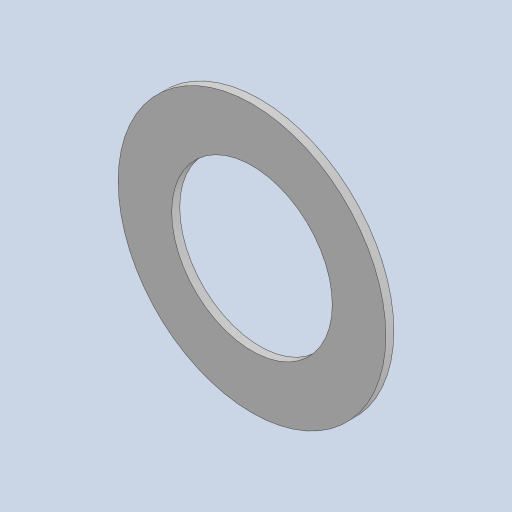
# Autodesk Inventor part: PACK-SWSJJ10-6-0_3
Saved by Autodesk Inventor 2023 (Build 270158000, 158)
## iProperties
Category: PARTsolutions
Company: MISUMI
Created: 2024-11-29
Part Number: PACK-SWSJJ10-6-0_3
Material: Generic
Catalog Web Link: www.cadenas.de
Description: SWSJJ, SWSJK, SWSPT, SWSPP, PACK-SWSJJ,PACK-SWSJK , PACK-SWSPT, PACK-SWSPP-Extra Thin Resin Washers / Sheets
Vendor: MISUMI
Document SubType Name: Modeling
Designer: psAdmin
Manufacturer: MISUMI
Mass: 0.0150796 g
Surface Area: 1.15611 cm^2
Volume: 0.0150796 cm^3
Density: 1 g/cm^3
Appearance: PSOLRGB-175-175-175
PSOL_IDENT_0: {$CADENAS_DATA/23d-libs/misumi/metric/26_washers_collars/swspt.prj},264 {VTYP=3D},{NB=PACK-SWSJJ10-6
PSOL_IDENT_1: -0.3},{LINA=PACK-SWSJJ10-6-0.3},{NN=SWSJJ, SWSJK, SWSPT, SWSPP, PACK-SWSJJ,PACK-SWSJK , PACK-SWSPT,
PSOL_IDENT_2: PACK-SWSPP},{DATE=15.11.2024 04:07:37},{GEOMDATE=13.04.2021 04:44:33},{VERSION=},{LINEID=10},{WBVAR=
PSOL_IDENT_3: COLOR,TYS,D,V,T},{WBNUMERIC=D,V,T}  {NB=PACK-SWSJJ10-6-0.3},{LINA=PACK-SWSJJ10-6-0.3},{KT=DUMMY},{PN=
PSOL_IDENT_4: PACK-SWSJJ10-6-0.3},{TYPE=SWSJJ},{MAT=Polyacetal},{MAT1=1},{COLOR=White},{COLORALG='White','White','
PSOL_IDENT_5: Black','Black'},{TYS=PACK-},{D=10},{DALG=8,10,12,14,15,16,20,25,30,35,40,50},{V=6},{VALG=0,3,4,5,6},
PSOL_IDENT_6: {T=0.3},{TALG=0.2,0.3,0.5,1.0},{TTOL=+/-0.04}
NB: PACK-SWSJJ10-6-0.3
NN: SWSJJ, SWSJK, SWSPT, SWSPP, PACK-SWSJJ,PACK-SWSJK , PACK-SWSPT, PACK-SWSPP
NT: Extra Thin Resin Washers / Sheets
NBSYN: $PN.
LINA: PACK-SWSJJ10-6-0.3
CATALOG: Misumi
PN: PACK-SWSJJ10-6-0.3
MAT: Polyacetal
COLOR: White
TYS: Washer Package
D: 10
V: 6
T: 0.3
TTOL: +/-0.04
SUPPLIER: MISUMI
ARTICLENO: PACK-SWSJJ10-6-0.3
BOMINFO: PACK-SWSJJ10-6-0.3
CREATOR: CADENAS GmbH
Title: PACK-SWSJJ10-6-0.3
Author: Cadenas PARTsolutions
Comments: Extra Thin Resin Washers / Sheets
Autodesk Inventor part; units mm, degrees
ref_plane "YZ Plane" through (0, 0, 0) normal (1, 0, 0) x (0, 1, 0)
ref_plane "XZ Plane" through (0, 0, 0) normal (0, 1, 0) x (-1, 0, 0)
ref_plane "XY Plane" through (0, 0, 0) normal (0, 0, 1) x (1, 0, 0)
sketch "Sketch_1" plane through (0, 0, 0) normal (0, 0, 1) x (1, 0, 0)
  circle A0 centre (0, 0) radius 5
  circle A1 centre (0, 0) radius 3
  dimension "d0" = 0.3
  constraints: 2 centre point
extrude "Extrusion1" add sketch "Sketch_1" along normal blind 0.3
body "Solid1"
